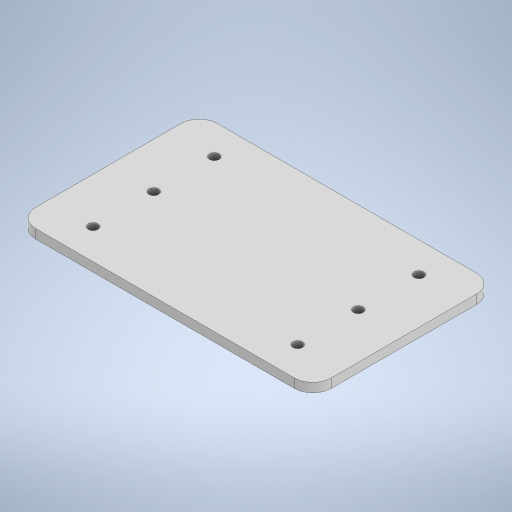
# Autodesk Inventor part: 足回り_固定
Saved by Autodesk Inventor 2023 (Build 270158000, 158)
## iProperties
Created: 2022-04-25
Part Number: 足回り_固定
Material: 一般
Document SubType Name: Modeling
Designer: yuta
Density: 1 g/cm^3
Appearance: 既定
Author: yuta
Autodesk Inventor part; units mm, degrees
ref_plane "YZ Plane" through (0, 0, 0) normal (1, 0, 0) x (0, 1, 0)
ref_plane "XZ Plane" through (0, 0, 0) normal (0, 1, 0) x (-1, 0, 0)
ref_plane "XY Plane" through (0, 0, 0) normal (0, 0, 1) x (1, 0, 0)
sketch "スケッチ1" plane through (0, 0, 0) normal (0, 1, 0) x (-1, 0, 0)
  line L0 (0, 0) -> (97.5, 0)
  line L1 (97.5, 0) -> (97.5, -60)
  line L2 (97.5, -60) -> (0, -60)
  line L3 (0, -60) -> (0, 0)
  dimension "d0" = 97.5
  dimension "d1" = 60
  constraints: 8 end point, 2 parallel, 1 horizontal, 1 perpendicular
  measures "d0" distance of L1.end L2.end
  measures "d1" distance of L0.end L1.end
extrude "押し出し1" add sketch "スケッチ1" along normal blind 3
sketch "スケッチ2" plane through (0, 3, 0) normal (0, 1, 0) x (1, 0, 0)
  line L0 (0, 0) -> (0, 60) projected
  line L1 (-97.5, 0) -> (0, 0) projected
  line L2 (-97.5, 60) -> (-97.5, 0) projected
  point P0 (-15, 30)
  point P1 (-15, 10)
  point P2 (-15, 50)
  point P3 (-82.5, 30)
  point P4 (-82.5, 10)
  point P5 (-82.5, 50)
  dimension "d4" = 15
  dimension "d5" = 30
  dimension "d6" = 20
  dimension "d7" = 20
  dimension "d8" = 15
  dimension "d9" = 15
  dimension "d10" = 15
  dimension "d11" = 15
  dimension "d12" = 15
  dimension "d13" = 20
  dimension "d14" = 20
  dimension "d15" = 30
  measures "d4" distance from line of L0 point (-15, 30)
  measures "d5" distance from line of L1 point (-15, 30)
  measures "d6" distance of point (-15, 10) point (-15, 30)
  measures "d7" distance of point (-15, 50) point (-15, 30)
  measures "d8" distance from line of L0 point (-15, 10)
  measures "d9" distance from line of L0 point (-15, 50)
  measures "d10" distance from line of point (-82.5, 30) L2
  measures "d11" distance from line of L2 point (-82.5, 10)
  measures "d12" distance from line of L2 point (-82.5, 50)
  measures "d13" distance of point (-82.5, 30) point (-82.5, 50)
  measures "d14" distance of point (-82.5, 30) point (-82.5, 10)
  measures "d15" distance from line of L1 point (-82.5, 30)
hole "穴1" at (-15, 3, -30) at (-15, 3, -10) at (-15, 3, -50) at (-82.5, 3, -30) at (-82.5, 3, -10) at (-82.5, 3, -50) direction (0, -1, 0) diameter 3.2 end through all
fillet "フィレット1" radius 6 4 edges at (-97.5, 1.5, 0) (0, 1.5, 0) (-97.5, 1.5, -60) (0, 1.5, -60)
